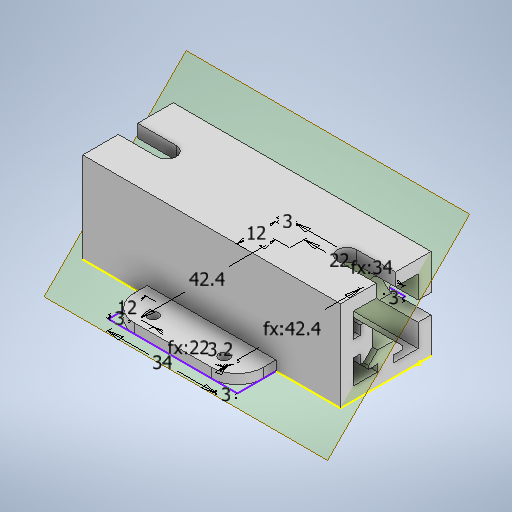
# Autodesk Inventor part: cameraSlider3
Saved by Autodesk Inventor 2025 (Build 290162000, 162)
## iProperties
Created: 2024-04-11
Part Number: cameraSlider3
Material: Generic
Document SubType Name: Modeling
Designer: cvss2
Density: 1 g/cm^3
Appearance: Default
Author: cvss2
Autodesk Inventor part; units mm, degrees
ref_plane "YZ Plane" through (0, 0, 0) normal (1, 0, 0) x (0, 1, 0)
ref_plane "XZ Plane" through (0, 0, 0) normal (0, 1, 0) x (-1, 0, 0)
ref_plane "XY Plane" through (0, 0, 0) normal (0, 0, 1) x (1, 0, 0)
sketch "Sketch1" plane through (0, 0, 0) normal (1, 0, 0) x (0, 1, 0)
  line L0 (0, 0) -> (20.1, 0)
  line L1 (20.1, 0) -> (20.1, 20.1)
  line L2 (20.1, 20.1) -> (0, 20.1)
  line L3 (0, 20.1) -> (0, 0)
  line L4 (-4, 24.1) -> (24.1, 24.1)
  line L5 (24.1, 24.1) -> (24.1, -4)
  line L6 (24.1, -4) -> (-4, -4)
  line L7 (-4, -4) -> (-4, 24.1)
  line L8 (12.55, 22.2) -> (7.55, 22.2)
  line L9 (7.55, 22.2) -> (7.55, 18)
  line L10 (7.55, 18) -> (12.55, 18)
  line L11 (12.55, 18) -> (12.55, 22.2)
  line L12 (12.55, 22.2) -> (7.55, 18) construction
  line L13 (7.55, 22.2) -> (12.55, 18) construction
  line L14 (12.55, 18) -> (15.35, 18)
  line L15 (15.35, 18) -> (15.35, 17)
  line L16 (15.35, 17) -> (12.55, 14.2)
  line L17 (12.55, 14.2) -> (7.55, 14.2)
  line L18 (7.55, 18) -> (4.75, 18)
  line L19 (4.75, 18) -> (4.75, 17)
  line L20 (4.75, 17) -> (7.55, 14.2)
  line L21 (2.1, 15.35) -> (3.1, 15.35)
  line L22 (3.1, 4.75) -> (5.9, 7.55)
  line L23 (2.1, 4.75) -> (3.1, 4.75)
  line L24 (-2.1, 12.55) -> (-2.1, 7.55)
  line L25 (2.1, 12.55) -> (-2.1, 12.55)
  line L26 (-2.1, 12.55) -> (2.1, 7.55) construction
  line L27 (-2.1, 7.55) -> (2.1, 12.55) construction
  line L28 (2.1, 7.55) -> (2.1, 4.75)
  line L29 (-2.1, 7.55) -> (2.1, 7.55)
  line L30 (2.1, 7.55) -> (2.1, 12.55)
  line L31 (5.9, 12.55) -> (5.9, 7.55)
  line L32 (2.1, 12.55) -> (2.1, 15.35)
  line L33 (3.1, 15.35) -> (5.9, 12.55)
  point P0 (10.05, 20.1)
  point P1 (0, 10.05)
  point P2 (10.05, 20.1)
  point P3 (0, 10.05)
  point P4 (0, 7.55)
  point P5 (0, 12.55)
  point P6 (7.55, 20.1)
  point P7 (12.55, 20.1)
  dimension "d0" = 20.1
  dimension "d1" = 20.1
  dimension "d2" = 4
  dimension "d3" = 5
  dimension "d4" = 4.2
  dimension "d5" = 2.8
  dimension "d6" = 1
  dimension "d7" = 3.8
  dimension "d8" = 2.8
  dimension "d9" = 5
  dimension "d10" = 1
  dimension "d11" = 135
  dimension "d12" = 5
  dimension "d13" = 4.2
  dimension "d14" = 2.8
  dimension "d15" = 1
  dimension "d16" = 3.8
  dimension "d17" = 2.8
  dimension "d18" = 5
  dimension "d19" = 1
  dimension "d20" = 135
  dimension "d21" = 7.55
  dimension "d22" = 2.1
  dimension "d23" = 90
  dimension "d24" = 7.55
  dimension "d25" = 2.1
  dimension "d26" = 90
  constraints: 68 end point, 10 parallel, 8 perpendicular, 6 midpoint, 1 horizontal, 3 other
  measures "d0" distance of L2.end L1.end
  measures "d1" distance of L1.end L0.end
  measures "d2" distance between parallel lines of L2 L4
  measures "d3" distance of L8.start L8.end
  measures "d4" distance of L12.end L8.end
  measures "d5" distance of L11.start L15.start
  measures "d6" distance of L15.start L15.end
  measures "d7" distance between parallel lines of L17 L14
  measures "d8" distance of L12.end L19.start
  measures "d9" distance of L17.start L20.end
  measures "d10" distance of L19.start L20.start
  measures "d11" angle of L17 L20
  measures "d12" distance of L24.start L24.end
  measures "d13" distance of L26.end L24.end
  measures "d14" distance of L25.start L32.end
  measures "d15" distance of L32.end L21.end
  measures "d16" distance between parallel lines of L31 L32
  measures "d17" distance of L26.end L28.end
  measures "d18" distance of L31.start L22.end
  measures "d19" distance of L28.end L23.end
  measures "d20" angle of L31 L22
  measures "d21" distance between parallel lines of L3 L9
  measures "d22" distance between parallel lines of L10 L2
  measures "d23" angle of L11 L14
  measures "d24" distance between parallel lines of L0 L29
  measures "d25" distance between parallel lines of L3 L28
  measures "d26" angle of L25 L32
extrude "Extrusion1" add sketch "Sketch1" against normal blind 80 contours L29 L24 L25 L3 | L3 L25 L30 L29 | L30 L32 L21 L33 L31 L22 L23 L28 | L11 L10 L9 L2 | L2 L9 L8 L11 | L14 L15 L16 L17 L20 L19 L18 L10 | L4 L5 L6 L7
sketch "Sketch2" plane through (0, -4, -4) normal (0, -1, 0) x (1, 0, 0)
  line L0 (0, 28.1) -> (0, 0) projected
  line L1 (0, 28.1) -> (-80, 28.1) projected
  line L2 (-80, 0) -> (-80, 28.1) projected
  line L3 (0, 0) -> (-80, 0) projected
  line L4 (-80, 0) -> (0, 28.1) construction
  line L5 (-80, 28.1) -> (0, 0) construction
  line L6 (-51, 35.25) -> (-51, -7.15) construction
  line L7 (-51, -7.15) -> (-29, -7.15) construction
  line L8 (-29, -7.15) -> (-29, 35.25) construction
  line L9 (-29, 35.25) -> (-51, 35.25) construction
  line L10 (-51, 35.25) -> (-29, -7.15) construction
  line L11 (-51, -7.15) -> (-29, 35.25) construction
  circle A0 centre (-29, 35.25) radius 1.6
  circle A1 centre (-29, -7.15) radius 1.6
  circle A2 centre (-51, 35.25) radius 1.6
  circle A3 centre (-51, -7.15) radius 1.6
  line L12 (-23, 28.1) -> (-57, 28.1)
  line L13 (-57, 40.1) -> (-23, 40.1)
  line L14 (-23, 0) -> (-57, 0)
  line L15 (-57, -12) -> (-23, -12)
  line L16 (-57, -12) -> (-60, -12)
  line L17 (-23, -12) -> (-20, -12)
  line L18 (-20, -12) -> (-20, 0)
  line L19 (-60, -12) -> (-60, 0)
  line L20 (-23, 40.1) -> (-20, 40.1)
  line L21 (-20, 40.1) -> (-20, 28.1)
  line L22 (0, 28.1) -> (-80, 28.1) projected
  line L23 (-57, 40.1) -> (-60, 40.1)
  line L24 (-60, 40.1) -> (-60, 28.1)
  point P0 (0, 4)
  point P1 (-40, 14.05)
  dimension "d29" = 42.4
  dimension "d31" = 22
  dimension "d32" = 3.2
  dimension "d35" = 42.4
  dimension "d38" = 22
  dimension "d41" = 34
  dimension "d42" = 12
  dimension "d44" = 12
  dimension "d46" = 34
  dimension "d59" = 3
  dimension "d60" = 3
  dimension "d61" = 3
  dimension "d62" = 3
  constraints: 40 end point, 8 point on line, 6 horizontal, 4 centre point, 4 coincident, 4 parallel, 4 perpendicular, 3 midpoint, 2 vertical, 9 other
  measures "d29" distance of L6.start L6.end
  measures "d31" distance of L7.end L6.end
  measures "d32" diameter of A0
  measures "d35" distance of L8.end point (-29, -7.15)
  measures "d38" distance of L8.end point (-51, 35.25)
  measures "d41" distance of L13.start L13.end
  measures "d42" distance of L12.end L13.start
  measures "d44" distance of L15.start L14.end
  measures "d46" distance of L15.start L15.end
  measures "d59" distance of L15.start L16.end
  measures "d60" distance of L15.end L17.end
  measures "d61" distance of L13.end L20.end
  measures "d62" distance of L13.start L23.end
extrude "Extrusion2" add sketch "Sketch2" against normal blind 3 contours L18 L17 L15 L16 L19 L3
sketch "Sketch3" plane through (0, 24.1, 24.1) normal (0, 1, 0) x (1, 0, 0)
  line L0 (0, 28.1) -> (0, 0) projected
  line L1 (0, 28.1) -> (-80, 28.1) projected
  line L2 (-80, 0) -> (-80, 28.1) projected
  line L3 (0, 0) -> (-80, 0) projected
  line L4 (0, 16.55) -> (0, 11.55) construction
  line L5 (0, 14.05) -> (-80, 14.05) construction
  line L6 (-80, 28.1) -> (-80, 0) construction
  circle A0 centre (-12, 14.05) radius 3
  circle A1 centre (-68, 14.05) radius 3
  line L7 (-68, 17.05) -> (-80, 17.05)
  line L8 (-68, 11.05) -> (-80, 11.05)
  line L9 (-12, 17.05) -> (0, 17.05)
  line L10 (0, 19.35) -> (0, 16.55) projected
  line L11 (-12, 11.05) -> (0, 11.05)
  line L12 (0, 8.75) -> (0, 11.55) projected
  point P0 (0, 24.1)
  point P1 (0, 11.05)
  point P2 (-80, 11.05)
  dimension "d49" = 6
  dimension "d50" = 6
  dimension "d51" = 12
  dimension "d52" = 12
  dimension "d53" = 6
  dimension "d54" = 6
  constraints: 10 end point, 6 point on line, 4 point on circle, 3 perpendicular, 2 centre point, 2 midpoint, 1 parallel
  measures "d49" diameter of A0
  measures "d50" diameter of A1
  measures "d51" distance from line of L2 A1.centre
  measures "d52" distance from line of L0 A0.centre
  measures "d53" distance between parallel lines of L11 L9
  measures "d54" distance between parallel lines of L8 L7
extrude "Extrusion3" cut sketch "Sketch3" against normal up to surface (4 mm away) contours L0 L11 A0 L9 | L7 A1 L8 L2 | A0 | A1
ref_plane "Work Plane1" through (0, 24.1, -4) normal (0, -0.7071068, -0.7071068) x (-1, 0, 0)
mirror "Mirror1" about plane through (0, 24.1, -4) normal (0, -0.7071068, -0.7071068) of "Extrusion3"
extrude "Extrusão4" add sketch "Sketch2" against normal blind 3 contours L1 L24 L23 L13 L20 L21
fillet "Arredondamento3" radius 8 4 edges at (-60, -2.5, 36.1) (-20, -2.5, 36.1) (-20, -2.5, -16) (-60, -2.5, -16)
equation "\"d8\" = d5"
equation "\"d9\" = d3"
equation "\"d10\" = d6"
equation "\"d17\" = d14"
equation "\"d18\" = d12"
equation "\"d19\" = d15"
body "Solid1"
